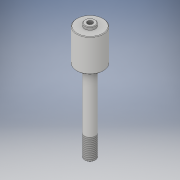
# Autodesk Inventor part: axe_rotation_principal
Saved by Autodesk Inventor 2019 (Build 230136000, 136)
## iProperties
Created: 2018-05-16
Part Number: axe_rotation_principal
Material: Générique
Document SubType Name: Modeling
Designer: Theo
Density: 1 g/cm^3
Appearance: Par défaut
Author: Theo
Autodesk Inventor part; units mm, degrees
ref_plane "YZ Plane" through (0, 0, 0) normal (1, 0, 0) x (0, 1, 0)
ref_plane "XZ Plane" through (0, 0, 0) normal (0, 1, 0) x (-1, 0, 0)
ref_plane "XY Plane" through (0, 0, 0) normal (0, 0, 1) x (1, 0, 0)
sketch "Esquisse1" plane through (0, 0, 0) normal (1, 0, 0) x (0, 1, 0)
  line L0 (2.5227, 0) -> (-2.5227, 0)
  line L1 (0, 5) -> (75.5, 5)
  line L2 (76, 8.5) -> (76, 12)
  line L3 (76, 12) -> (76.5, 12.5)
  line L4 (76.5, 12.5) -> (106, 12.5)
  line L5 (0, 5) -> (0, 0)
  line L6 (0, 0) -> (109.25, 0)
  line L7 (106.5, 5) -> (106.5, 12)
  line L8 (106, 12.5) -> (106.5, 12)
  line L9 (76, 8.5) -> (75.5, 7.5)
  line L10 (75.5, 7.5) -> (75.5, 5)
  line L11 (109.25, 0) -> (109.25, 4.5)
  line L12 (109.25, 4.5) -> (108.75, 5)
  line L13 (108.75, 5) -> (106.5, 5)
  dimension "d2" = 0.5
  dimension "d3" = 0.5
  dimension "d6" = 10
  dimension "d7" = 76
  dimension "d8" = 25
  dimension "d9" = 0.5
  dimension "d10" = 0.5
  dimension "d11" = 30.5
  dimension "d13" = 1
  dimension "d14" = 0.5
  dimension "d15" = 17
  dimension "d23" = 0.5
  dimension "d24" = 0.5
  dimension "d25" = 10
  dimension "d26" = 2.75
  constraints: 28 end point, 5 horizontal, 5 vertical, 1 coincident, 1 midpoint
  measures "d2" horizontal distance of L2.end L3.end
  measures "d3" horizontal distance of L2.end L3.end
  measures "d6" diameter of L1 L0
  measures "d7" distance between parallel lines of L2 L5
  measures "d8" diameter of L4 L0
  measures "d9" horizontal distance of L4.end L7.end
  measures "d10" horizontal distance of L4.end L7.end
  measures "d11" distance between parallel lines of L7 L2
  measures "d13" vertical distance of L2.start L9.end
  measures "d14" horizontal distance of L2.start L9.end
  measures "d15" diameter of L2.start L0
  measures "d23" horizontal distance of L11.end L12.end
  measures "d24" horizontal distance of L11.end L12.end
  measures "d25" diameter of L13 L0
  measures "d26" distance between parallel lines of L11 L7
revolve "Révolution1" add sketch "Esquisse1" angle 360 about axis through (0, 2.5227, 0) along (0, -1, 0)
thread "Filetage2" size "M10x1.5" class "6g" standard "ISO Metric profile" length 20
chamfer "Chanfrein1" distance 0.5 angle 45 1 edges at (0, 0, -5)
sketch "Esquisse4" plane through (0, 109.25, 0) normal (0, 1, 0) x (1, 0, 0)
  circle A0 centre (0, 0) radius 4.5 projected
  point P0 (0, 0)
  constraints: 1 coincident
hole "Perçage2" at (0, 109.25, 0) direction (0, -1, 0) diameter 4.917 depth 17.1 tip angle 118 thread size "M6x1" class "6H" standard "ISO Metric profile"
equation "\"d3\" = d2"
equation "\"d10\" = d9"
equation "\"d24\" = d23"
